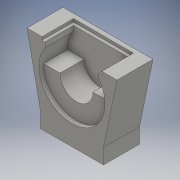
# Autodesk Inventor part: main-base
Saved by Autodesk Inventor 2016 (Build 200138000, 138)
## iProperties
Created: 2016-10-30
Part Number: main-base
Material: Generic
Document SubType Name: Modeling
Designer: Matt Ruffner
Density: 1 g/cm^3
Appearance: Default
Author: Matt Ruffner
Autodesk Inventor part; units mm, degrees
ref_plane "YZ Plane" through (0, 0, 0) normal (1, 0, 0) x (0, 1, 0)
ref_plane "XZ Plane" through (0, 0, 0) normal (0, 1, 0) x (-1, 0, 0)
ref_plane "XY Plane" through (0, 0, 0) normal (0, 0, 1) x (1, 0, 0)
sketch "Sketch1" plane through (0, 0, 0) normal (1, 0, 0) x (0, 1, 0)
  arc A0 (11.6517, 2.8247) -> (11.6517, -22.0843) centre (-6.4834, -9.6298) ccw
  line L0 (11.6517, 20.3702) -> (11.6517, 2.8247)
  line L1 (11.6517, -22.0843) -> (11.6517, -39.6298)
  line L2 (11.6517, -39.6298) -> (-31.884, -30.6298)
  line L3 (-31.884, -30.6298) -> (-31.884, 11.3702)
  line L4 (-31.884, 11.3702) -> (11.6517, 20.3702)
  line L5 (11.6517, 2.8247) -> (11.6517, -22.0843)
  point P0 (0, 0)
  dimension "d4" = 44
  dimension "d5" = 60
  dimension "d6" = 30
  dimension "d7" = 42
  dimension "d8" = 9
  constraints: 12 end point, 4 vertical, 2 point on circle, 1 centre point, 1 coincident
  measures "d4" diameter of A0
  measures "d5" distance of L0.start L1.end
  measures "d6" vertical distance of A0.centre L1.end
  measures "d7" distance of L2.end L3.end
  measures "d8" vertical distance of L0.start L3.end
extrude "Extrusion1" add sketch "Sketch1" along normal blind 24
shell "Shell1" thickness 3 removed faces 1 at (8, 11.6517, -19.6298)
sketch "Sketch2" plane through (24, 0, 0) normal (1, 0, 0) x (0, 0, -1)
  arc A0 (-8.3702, 6.3008) -> (27.6298, 6.3008) centre (9.6298, -6.3483) ccw
  line L0 (39.6298, 11.6517) -> (-20.3702, 11.6517) projected
  line L1 (-20.3702, 11.6517) -> (-11.3702, -31.884) projected
  line L2 (-11.3702, -31.884) -> (30.6298, -31.884) projected
  line L3 (30.6298, -31.884) -> (39.6298, 11.6517) projected
  line L4 (39.6298, 11.6517) -> (-20.3702, 11.6517) projected
  line L5 (-8.3702, 11.6517) -> (-8.3702, 6.3008)
  line L6 (27.6298, 11.6517) -> (27.6298, 6.3008)
  point P0 (0, 0)
  dimension "d14" = 44
  dimension "d16" = 12
  dimension "d17" = 30
  dimension "d18" = 12
  constraints: 4 end point, 2 point on circle, 2 point on line, 1 centre point, 1 perpendicular, 1 vertical
  measures "d14" diameter of A0
  measures "d16" distance of L0.end L5.start
  measures "d17" horizontal distance of L0.end A0.centre
  measures "d18" distance of L0.start L6.start
extrude "Extrusion2" cut sketch "Sketch2" against normal up to next contours L5 L0 L6 A0
sketch "Sketch3" plane through (0, -31.884, -30.6298) normal (0, -1, 0) x (1, 0, 0)
  line L0 (0, 42) -> (0, 0) projected
  line L1 (0, 0) -> (24, 0) projected
  line L2 (24, 42) -> (24, 0) projected
  line L3 (0, 42) -> (24, 42) projected
  point P0 (0, 30.6298)
extrude "Extrusion3" add sketch "Sketch3" along normal blind 10
sketch "Sketch4" plane through (21, -28.884, -28.1866) normal (-1, 0, 0) x (0, 0, 1)
  line L0 (0.5567, 35.1848) -> (0.5567, 40.5357) projected
  line L1 (-8.3798, 40.5357) -> (0.5567, 40.5357) projected
  line L2 (0, 0) -> (-8.3798, 40.5357) projected
  line L3 (37.1135, 0) -> (0, 0) projected
  line L4 (45.4933, 40.5357) -> (37.1135, 0) projected
  line L5 (36.5567, 40.5357) -> (45.4933, 40.5357) projected
  line L6 (36.5567, 40.5357) -> (36.5567, 35.1848) projected
  arc A0 (0.5567, 35.1848) -> (36.5567, 35.1848) centre (18.5567, 22.5357) ccw projected
  arc A1 (7.5567, 22.5357) -> (29.5567, 22.5357) centre (18.5567, 22.5357) ccw
  line L7 (7.5567, 22.5357) -> (-3.4433, 22.5357)
  line L8 (29.5567, 22.5357) -> (40.5567, 22.5357)
  point P0 (28.1866, 28.884)
  dimension "d23" = 22
  constraints: 4 end point, 4 point on circle, 2 point on line, 1 centre point, 1 coincident, 1 horizontal
  measures "d23" diameter of A1
extrude "Extrusion4" add sketch "Sketch4" along normal up to next
sketch "Sketch5" plane through (0, 11.6517, -39.6298) normal (0, 1, 0) x (1, 0, 0)
  line L0 (3, -50) -> (21, -50)
  line L1 (21, -50) -> (21, -10)
  line L2 (21, -10) -> (3, -10)
  line L3 (3, -10) -> (3, -50)
  line L4 (0, -60) -> (24, -60) projected
  line L5 (0, 0) -> (0, -60) projected
  point P0 (0, -39.6298)
  dimension "d26" = 40
  dimension "d27" = 10
  dimension "d28" = 18
  dimension "d29" = 3
  constraints: 8 end point, 2 parallel, 1 horizontal, 1 perpendicular
  measures "d26" distance between parallel lines of L2 L0
  measures "d27" distance between parallel lines of L4 L0
  measures "d28" distance of L0.start L0.end
  measures "d29" distance between parallel lines of L5 L3
sketch "Sketch6" plane through (3, 6.3008, 8.3702) normal (1, 0, 0) x (0, 0, -1)
  line L0 (0, 5.3509) -> (0, 0) projected
  arc A0 (0, 0) -> (-4, -12.6491) centre (18, -12.6491) ccw projected
  line L1 (-4, -12.6491) -> (7, -12.6491) projected
  arc A1 (7, -12.6491) -> (29, -12.6491) centre (18, -12.6491) ccw projected
  line L2 (29, -12.6491) -> (40, -12.6491) projected
  arc A2 (40, -12.6491) -> (36, 0) centre (18, -12.6491) ccw projected
  line L3 (36, 0) -> (36, 5.3509) projected
  line L4 (0, 5.3509) -> (36, 5.3509) projected
  point P0 (8.3702, -6.3008)
extrude "Extrusion5" add sketch "Sketch6" along normal blind 2
extrude "Extrusion6" cut sketch "Sketch5" against normal blind 2
sketch "Sketch7" plane through (21, 11.6517, -29.6298) normal (-1, 0, 0) x (0, 0, 1)
  line L0 (2, 0) -> (2, -2) projected
  line L1 (0, 0) -> (2, 0) projected
  line L2 (0, 0) -> (0, -2) projected
  line L3 (0, -2) -> (2, -2) projected
  line L4 (38, -2) -> (38, 0) projected
  line L5 (38, -2) -> (40, -2) projected
  line L6 (40, 0) -> (40, -2) projected
  line L7 (38, 0) -> (40, 0) projected
  point P0 (29.6298, -11.6517)
extrude "Extrusion7" cut sketch "Sketch7" against normal up to next contours L0 L3 L2 L1
sketch "Sketch8" plane through (21, 11.6517, 8.3702) normal (-1, 0, 0) x (0, 0, 1)
  line L0 (0, -2) -> (0, 0) projected
  line L1 (0, -2) -> (2, -2) projected
  line L2 (2, 0) -> (2, -2) projected
  line L3 (0, 0) -> (2, 0) projected
  point P0 (-8.3702, -11.6517)
extrude "Extrusion8" cut sketch "Sketch8" against normal up to next
body "Solid1"
